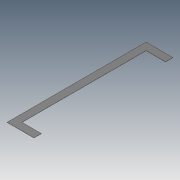
# Autodesk Inventor part: Panel_E
Saved by Autodesk Inventor 2020 (Build 240168000, 168)
## iProperties
Created: 2021-02-24
Part Number: Panel_E
Material: アルミニウム 6061
Document SubType Name: Modeling
Designer: magnarecta
Density: 2.7 g/cm^3
Appearance: 細かい テクスチャ - 黒
Author: magnarecta
Autodesk Inventor part; units mm, degrees
ref_plane "YZ Plane" through (0, 0, 0) normal (1, 0, 0) x (0, 1, 0)
ref_plane "XZ Plane" through (0, 0, 0) normal (0, 1, 0) x (-1, 0, 0)
ref_plane "XY Plane" through (0, 0, 0) normal (0, 0, 1) x (1, 0, 0)
sketch "スケッチ1" plane through (0, 0, 0) normal (0, 1, 0) x (-1, 0, 0)
  line L0 (-145, -750) -> (145, -750)
  line L1 (145, -750) -> (145, 750)
  line L2 (145, 750) -> (-145, 750)
  line L3 (-145, 750) -> (-145, -750)
  line L4 (-145, -750) -> (145, 750) construction
  line L5 (145, -750) -> (-145, 750) construction
  point P0 (0, 0)
  dimension "d0" = 1500
  dimension "d1" = 290
  constraints: 12 end point, 2 midpoint, 2 parallel, 1 horizontal, 1 perpendicular
  measures "d0" distance of L0.end L1.end
  measures "d1" distance of L1.end L2.end
extrude "押し出し1" add sketch "スケッチ1" along normal blind 2
sketch "スケッチ2" plane through (0, 2, 0) normal (0, 1, 0) x (1, 0, 0)
  line L0 (355, 670) -> (-65, 670)
  line L1 (-65, 670) -> (-65, -670)
  line L2 (-65, -670) -> (355, -670)
  line L3 (355, -670) -> (355, 670)
  line L4 (145, -750) -> (145, 750) projected
  line L5 (355, 670) -> (-65, -670) construction
  line L6 (-65, 670) -> (355, -670) construction
  line L7 (-145, -750) -> (145, -750) projected
  line L8 (-145, 750) -> (-145, -750) projected
  point P0 (0, 0)
  point P1 (145, 0)
  point P2 (145, -670)
  point P3 (145, 670)
  dimension "d4" = 80
  dimension "d5" = 80
  constraints: 12 end point, 3 midpoint, 2 parallel, 1 horizontal, 1 perpendicular
  measures "d4" distance between parallel lines of L7 L2
  measures "d5" distance between parallel lines of L8 L1
extrude "押し出し2" cut sketch "スケッチ2" against normal blind 10 contours L4 L2 L1 L0
